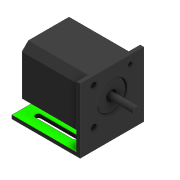
# Autodesk Inventor part: Nema 17 CNC Kit Stepper Motor
Saved by Autodesk Inventor 2020 (Build 240168000, 168)
## iProperties
Created: 2021-03-06
Part Number: Nema 17 CNC Kit Stepper Motor
Material: Generic
Document SubType Name: Modeling
Designer: Coy
Density: 1 g/cm^3
Appearance: Default(1)
Author: Coy
Autodesk Inventor part; units mm, degrees
ref_plane "YZ Plane" through (0, 0, 0) normal (1, 0, 0) x (0, 1, 0)
ref_plane "XZ Plane" through (0, 0, 0) normal (0, 1, 0) x (-1, 0, 0)
ref_plane "XY Plane" through (0, 0, 0) normal (0, 0, 1) x (1, 0, 0)
sketch "Sketch1" plane through (0, 0, 0) normal (1, 0, 0) x (0, 1, 0)
  line L0 (0, 0) -> (42, 0)
  line L1 (42, 0) -> (42, 42)
  line L2 (42, 42) -> (0, 42)
  line L3 (0, 42) -> (0, 0)
  dimension "d0" = 42
  dimension "d1" = 42
  constraints: 8 end point, 2 parallel, 1 horizontal, 1 perpendicular
  measures "d0" distance of L2.end L1.end
  measures "d1" distance of L1.end L0.end
extrude "Extrusion1" add sketch "Sketch1" against normal blind 47
sketch "Sketch2" plane through (0, 0, 0) normal (1, 0, 0) x (0, 0, -1)
  line L0 (-42, 42) -> (0, 42) construction
  line L1 (-21, 42) -> (-21, 0) construction
  line L2 (0, 0) -> (-42, 0) construction
  circle A0 centre (-21, 21) radius 11
  circle A1 centre (-21, 21) radius 4
  dimension "d4" = 22
  dimension "d5" = 8
  constraints: 3 midpoint, 2 centre point, 2 end point, 1 coincident
  measures "d4" diameter of A0
  measures "d5" diameter of A1
extrude "Extrusion2" add sketch "Sketch2" along normal blind 2
sketch "Sketch3" plane through (0, 21, 21) normal (1, 0, 0) x (0, 0, -1)
  circle A0 centre (0, 0) radius 4 projected
  circle A1 centre (0, 0) radius 2.5
  point P0 (21, -21)
  dimension "d8" = 5
  constraints: 1 centre point, 1 coincident
  measures "d8" diameter of A1
extrude "Extrusion3" add sketch "Sketch3" along normal blind 22 contours A1
chamfer "Chamfer1" distance 5 angle 45 4 edges at (-23.5, 42, 42) (-23.5, 42, 0) (-23.5, 0, 42) (-23.5, 0, 0)
sketch "Sketch4" plane through (0, 0, 0) normal (1, 0, 0) x (0, 0, -1)
  line L0 (-35.375, 35.3745) -> (-6.625, 35.3745) construction
  line L1 (-6.625, 35.3745) -> (-6.625, 6.6245) construction
  line L2 (-6.625, 6.6245) -> (-35.375, 6.6245) construction
  line L3 (-35.375, 6.6245) -> (-35.375, 35.3745) construction
  line L4 (-42, 37) -> (-42, 5) construction
  line L5 (-5, 42) -> (-37, 42) construction
  circle A0 centre (-6.625, 35.3745) radius 1.25
  circle A1 centre (-35.375, 35.3745) radius 1.25
  circle A2 centre (-35.375, 6.6245) radius 1.25
  circle A3 centre (-6.625, 6.6245) radius 1.25
  point P0 (0, 0)
  dimension "d14" = 28.75
  dimension "d15" = 28.75
  dimension "d16" = 6.625
  dimension "d17" = 6.6255
  dimension "d18" = 2.5
  dimension "d19" = 2.5
  dimension "d20" = 2.5
  dimension "d21" = 2.5
  constraints: 8 end point, 4 centre point, 4 coincident, 2 parallel, 1 horizontal, 1 perpendicular
  measures "d14" distance of L1.end L2.end
  measures "d15" distance of L0.end L1.end
  measures "d16" distance between parallel lines of L4 L3
  measures "d17" distance between parallel lines of L5 L0
  measures "d18" diameter of A0
  measures "d19" diameter of A1
  measures "d20" diameter of A2
  measures "d21" diameter of A3
extrude "Extrusion4" cut sketch "Sketch4" against normal blind 5
sketch "Sketch5" plane through (0, 0, 0) normal (1, 0, 0) x (0, 0, -1)
  line L0 (-46, 42) -> (4, 42)
  line L1 (4, 42) -> (4, -9)
  line L2 (4, -9) -> (-46, -9)
  line L3 (-46, -9) -> (-46, 42)
  line L4 (-5, 42) -> (-37, 42) construction
  line L5 (-42, 37) -> (-42, 5) construction
  circle A0 centre (-21, 21) radius 11 projected
  circle A1 centre (-35.375, 35.3745) radius 1.25 projected
  circle A2 centre (-6.625, 35.3745) radius 1.25 projected
  circle A3 centre (-6.625, 6.6245) radius 1.25 projected
  circle A4 centre (-35.375, 6.6245) radius 1.25 projected
  circle A5 centre (-35.375, 35.3745) radius 2.3338
  circle A6 centre (-6.625, 35.3745) radius 1.7372
  circle A7 centre (-35.375, 6.6245) radius 2.4239
  circle A8 centre (-6.625, 6.6245) radius 2.2788
  circle A9 centre (-21, 21) radius 12
  point P0 (0, 0)
  dimension "d24" = 50
  dimension "d25" = 51
  dimension "d26" = 4
  dimension "d27" = 0
  dimension "d28" = 1.0838
  dimension "d29" = 0.4872
  dimension "d30" = 1.1739
  dimension "d31" = 1.0288
  dimension "d32" = 1
  constraints: 8 end point, 5 centre point, 2 parallel, 1 horizontal, 1 perpendicular
  measures "d24" distance of L1.end L2.end
  measures "d25" distance of L0.end L1.end
  measures "d26" distance between parallel lines of L5 L3
  measures "d27" distance between parallel lines of L4 L0
  measures "d28" radial gap between concentric circles of A1 A5
  measures "d29" radial gap between concentric circles of A2 A6
  measures "d30" radial gap between concentric circles of A4 A7
  measures "d31" radial gap between concentric circles of A3 A8
  measures "d32" radial gap between concentric circles of A0 A9
extrude "Extrusion5" add sketch "Sketch5" along normal blind 2.75 contours L0 L1 L2 L3
sketch "Sketch6" plane through (0, 0, 0) normal (-1, 0, 0) x (0, 0, 1)
  line L0 (42, 37) -> (37, 42) projected
  line L1 (42, 37) -> (42, 5) projected
  line L2 (37, 0) -> (42, 5) projected
  line L3 (37, 0) -> (5, 0) projected
  line L4 (0, 5) -> (5, 0) projected
  line L5 (0, 5) -> (0, 37) projected
  line L6 (5, 42) -> (0, 37) projected
  line L7 (-4, 42) -> (5, 42) projected
  line L8 (-4, -9) -> (-4, 42) projected
  line L9 (46, -9) -> (-4, -9) projected
  line L10 (46, 42) -> (46, -9) projected
  line L11 (37, 42) -> (46, 42) projected
  line L12 (-4, -6.25) -> (46, -6.25)
  line L13 (46, 42) -> (46, -9) projected
  point P0 (0, 0)
  dimension "d35" = 2.75
  constraints: 2 end point, 2 point on line, 1 perpendicular
  measures "d35" distance between parallel lines of L9 L12
extrude "Extrusion6" add sketch "Sketch6" along normal blind 51 contours L10 L9 L8 L12
sketch "Sketch7" plane through (2.75, -9, -4) normal (0, -1, 0) x (1, 0, 0)
  line L0 (-42.625, 9.625) -> (-13.625, 9.625) construction
  line L1 (-42.625, 7.5) -> (-13.625, 7.5)
  line L2 (-13.625, 11.75) -> (-42.625, 11.75)
  arc A0 (-42.625, 11.75) -> (-42.625, 7.5) centre (-42.625, 9.625) ccw
  arc A1 (-13.625, 7.5) -> (-13.625, 11.75) centre (-13.625, 9.625) ccw
  line L3 (-53.75, 0) -> (0, 0) projected
  line L4 (-53.75, 0) -> (-53.75, 50) projected
  line L5 (-53.75, 25) -> (0, 25) construction
  line L6 (0, 50) -> (0, 0) construction
  line L7 (-42.625, 42.5) -> (-13.625, 42.5)
  line L8 (-13.625, 38.25) -> (-42.625, 38.25)
  arc A2 (-42.625, 42.5) -> (-42.625, 38.25) centre (-42.625, 40.375) ccw
  arc A3 (-13.625, 38.25) -> (-13.625, 42.5) centre (-13.625, 40.375) ccw
  point P0 (-2.75, 4)
  point P1 (-28.125, 9.625)
  dimension "d38" = 29
  dimension "d39" = 4.25
  dimension "d40" = 7.5
  dimension "d41" = 11.125
  constraints: 14 end point, 8 point on circle, 6 symmetric about line, 4 centre point, 4 tangent, 3 midpoint, 1 horizontal, 1 parallel, 2 other
  measures "d38" distance of L0.start L0.end
  measures "d39" diameter of A1
  measures "d40" distance between parallel lines of L3 L1
  measures "d41" distance from line of L4 L0.start
extrude "Extrusion7" cut sketch "Sketch7" against normal up to next
body "Solid1"
